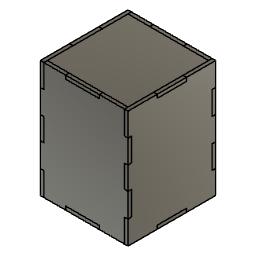
box v1 (1) (Autodesk Fusion 360 design; units mm, degrees)
Autodesk Fusion 360 part; units mm, degrees
sketch "base" plane through (0, 0, 0) normal (0, 0, 1) x (1, 0, 0)
  line L0 (37.5, 37.5) -> (-37.5, 37.5)
  line L1 (-37.5, 37.5) -> (-37.5, -37.5)
  line L2 (-37.5, -37.5) -> (37.5, -37.5)
  line L3 (37.5, -37.5) -> (37.5, 37.5)
  line L4 (37.5, 37.5) -> (-37.5, -37.5) construction
  line L5 (-37.5, 37.5) -> (37.5, -37.5) construction
  dimension "d7" = 75
  dimension "d8" = 75
  constraint horizontal L0
  constraint perpendicular L0 L1
  constraint parallel L0 L2
  constraint parallel L1 L3
  constraint coincident L4 origin
  constraint coincident L5 origin
  measures "d7" distance of L1.end L2.end
  measures "d8" distance of L0.end L1.end
extrude "Extrude1" add sketch "base" along normal blind 3 makes body 1
sketch "Sketch3" plane through (0, -37.5, 0) normal (0, -1, 0) x (1, 0, 0)
  line L0 (-37.5, 0) -> (37.5, 0)
  line L1 (37.5, 0) -> (37.5, 3)
  line L2 (37.5, 3) -> (-37.5, 3)
  line L3 (-37.5, 3) -> (-37.5, 0)
  line L4 (-37.5, 0) -> (37.5, 0)
  line L5 (37.5, 0) -> (37.5, 100)
  line L6 (37.5, 100) -> (-37.5, 100)
  line L7 (-37.5, 100) -> (-37.5, 0)
  line L8 (-15.7952, 3) -> (13, 3)
  line L9 (13, 3) -> (13, 0)
  line L10 (13, 0) -> (-15.7952, 0)
  line L11 (-15.7952, 0) -> (-15.7952, 3)
  dimension "d11" = 100
  constraint perpendicular L4 L5
  constraint parallel L4 L6
  constraint parallel L5 L7
  constraint coincident L0.end L1.start
  constraint perpendicular L1 L4
  constraint coincident L0.start L3.end
  constraint horizontal L8
  constraint vertical L9
  constraint horizontal L10
  constraint vertical L11
  constraint coincident L4 L9.end
  constraint coincident L2 L8.start
  measures "d11" distance of L0.start L6.end
extrude "Extrude3" add sketch "Sketch3" against normal blind 3 separate body contours L0 L2 L3 L4 L7 L11 | L2 L5 L6 L7 L8 | L0 L1 L2 L4 L5 L9 makes body 2
extrude "Extrude4" add 1 faces at (4.3333, -34.5, 67.6667) along direction (0, -1, 0) blind 3 from surface at -72 separate body on bodies 2 makes body 3
combine "Combine1" operation cut target body 1 tool bodies 3 2 keep tools
sketch "Sketch5" plane through (-37.5, 0, 0) normal (-1, 0, 0) x (0, -1, 0)
  line L0 (34.5, 0) -> (34.5, 3)
  line L1 (34.5, 3) -> (-34.5, 3)
  line L2 (-34.5, 3) -> (-34.5, 0)
  line L3 (-34.5, 0) -> (34.5, 0)
  line L4 (-37.5, 100) -> (-37.5, 0)
  line L5 (-37.5, 0) -> (-34.5, 0)
  line L6 (-34.5, 0) -> (-34.5, 100)
  line L7 (-34.5, 100) -> (-37.5, 100)
  line L8 (37.5, 0) -> (37.5, 100)
  line L9 (37.5, 100) -> (34.5, 100)
  line L10 (34.5, 100) -> (34.5, 0)
  line L11 (34.5, 0) -> (37.5, 0)
  line L12 (-37.5, 100) -> (37.5, 100)
  line L13 (37.5, 100) -> (37.5, 0)
  line L14 (37.5, 0) -> (-37.5, 0)
  line L15 (-37.5, 0) -> (-37.5, 100)
  line L16 (-37.5, 80) -> (-34.5, 80)
  line L17 (-34.5, 80) -> (-34.5, 60)
  line L18 (-34.5, 60) -> (-37.5, 60)
  line L19 (-37.5, 60) -> (-37.5, 80)
  line L20 (-37.5, 56.4805) -> (-37.5, 40)
  line L21 (34.5, 80) -> (37.5, 80)
  line L22 (37.5, 80) -> (37.5, 60)
  line L23 (37.5, 60) -> (34.5, 60)
  line L24 (34.5, 60) -> (34.5, 80)
  line L25 (34.5, 20) -> (37.5, 20)
  line L26 (37.5, 20) -> (37.5, 40)
  line L27 (37.5, 40) -> (34.5, 40)
  line L28 (34.5, 40) -> (34.5, 20)
  line L29 (12.5, 3) -> (-12.5, 3)
  line L30 (-12.5, 3) -> (-12.5, 0)
  line L31 (-12.5, 0) -> (12.5, 0)
  line L32 (12.5, 0) -> (12.5, 3)
  line L33 (37.5, 40.56) -> (34.5, 40.56)
  line L34 (34.5, 40.56) -> (34.5, 25)
  line L35 (34.5, 25) -> (37.5, 25)
  line L36 (37.5, 25) -> (37.5, 40.56)
  line L37 (-37.5, 39.7052) -> (-34.5, 39.7052)
  line L38 (-34.5, 39.7052) -> (-34.5, 20)
  line L39 (-34.5, 20) -> (-37.5, 20)
  line L40 (-37.5, 20) -> (-37.5, 39.7052)
  dimension "d25" = 20
  dimension "d26" = 20
  dimension "d28" = 20
  dimension "d31" = 20
  dimension "d33" = 25
  dimension "d36" = 25
  dimension "d37" = 20
  dimension "d39" = 20
  dimension "d40" = 20
  dimension "d41" = 20
  constraint horizontal L12
  constraint vertical L13
  constraint horizontal L14
  constraint vertical L15
  constraint coincident L8.start L11.end
  constraint coincident L4.start L7.end
  constraint horizontal L16
  constraint vertical L17
  constraint horizontal L18
  constraint vertical L19
  constraint coincident L6 L17.end
  constraint coincident L15 L16.start
  constraint vertical L20
  constraint coincident L4 L20.end
  constraint horizontal L21
  constraint vertical L22
  constraint horizontal L23
  constraint vertical L24
  constraint coincident L13 L22.end
  constraint coincident L10 L21.start
  constraint horizontal L25
  constraint vertical L26
  constraint horizontal L27
  constraint vertical L28
  constraint coincident L8 L26.end
  constraint coincident L10 L25.start
  constraint horizontal L29
  constraint vertical L30
  constraint horizontal L31
  constraint vertical L32
  constraint coincident L14 L30.end
  constraint coincident L1 L29.start
  constraint horizontal L33
  constraint vertical L34
  constraint horizontal L35
  constraint vertical L36
  constraint coincident L10 L34.end
  constraint coincident L13 L33.start
  constraint horizontal L37
  constraint vertical L38
  constraint horizontal L39
  constraint vertical L40
  constraint coincident L6 L38.end
  constraint coincident L20 L37.start
  measures "d25" distance of L8.end L21.end
  measures "d26" distance of L21.start L23.end
  measures "d28" distance of L4.start L16.start
  measures "d31" distance of L16.start L18.end
  measures "d33" distance of L8.start L31.end
  measures "d36" distance of L29.start L29.end
  measures "d37" distance of L22.end L26.end
  measures "d39" distance of L18.end L20.end
  measures "d40" distance of L20.end L39.end
  measures "d41" distance of L25.end L26.end
extrude "Extrude5" add sketch "Sketch5" against normal blind 3 separate body contours L0 L1 L3 L10 L14 L32 | L0 L8 L10 L11 L13 L14 L25 | L1 L6 L10 L12 L17 L24 L28 L29 L34 L38 | L1 L2 L3 L6 L14 L30 | L2 L4 L5 L6 L14 L15 L39 | L8 L10 L13 L23 L33 | L4 L6 L15 L18 L20 L37 | L8 L9 L10 L12 L13 L21 | L4 L6 L7 L12 L15 L16 makes body 4
extrude "Extrude6" add 1 faces at (-34.5, -4.1667, 27.5684) along direction (-1, 0, 0) blind 3 from surface at -72 separate body on bodies 4 makes body 5
combine "Combine2" operation cut target body 2 tool bodies 5 4 keep tools
sketch "Sketch7" plane through (0, 37.5, 0) normal (0, 1, 0) x (-1, 0, 0)
  line L0 (-13, 3) -> (15.7952, 3)
  line L1 (15.7952, 3) -> (15.7952, 0)
  line L2 (15.7952, 0) -> (37.5, 0)
  line L3 (37.5, 0) -> (37.5, 100)
  line L4 (37.5, 100) -> (-37.5, 100)
  line L5 (-37.5, 100) -> (-37.5, 0)
  line L6 (-37.5, 0) -> (-13, 0)
  line L7 (-13, 0) -> (-13, 3)
combine "Combine3" operation cut target body 3 tool bodies 5 4 keep tools
sketch "Sketch8" plane through (0, -37.5, 0) normal (0, -1, 0) x (1, 0, 0)
  line L0 (-34.5, 20) -> (-34.5, 0)
  line L1 (-34.5, 0) -> (-15.7952, 0)
  line L2 (-15.7952, 0) -> (-15.7952, 3)
  line L3 (-15.7952, 3) -> (13, 3)
  line L4 (13, 3) -> (13, 0)
  line L5 (13, 0) -> (34.5, 0)
  line L6 (34.5, 0) -> (34.5, 20)
  line L7 (34.5, 20) -> (37.5, 20)
  line L8 (37.5, 20) -> (37.5, 40.56)
  line L9 (37.5, 40.56) -> (34.5, 40.56)
  line L10 (34.5, 40.56) -> (34.5, 60)
  line L11 (34.5, 60) -> (37.5, 60)
  line L12 (37.5, 60) -> (37.5, 80)
  line L13 (37.5, 80) -> (34.5, 80)
  line L14 (34.5, 80) -> (34.5, 100)
  line L15 (34.5, 100) -> (-34.5, 100)
  line L16 (-34.5, 100) -> (-34.5, 80)
  line L17 (-34.5, 80) -> (-37.5, 80)
  line L18 (-37.5, 80) -> (-37.5, 60)
  line L19 (-37.5, 60) -> (-34.5, 60)
  line L20 (-34.5, 60) -> (-34.5, 40.56)
  line L21 (-34.5, 40.56) -> (-37.5, 40.56)
  line L22 (-37.5, 40.56) -> (-37.5, 20)
  line L23 (-37.5, 20) -> (-34.5, 20)
sketch "Sketch9" plane through (0, -37.5, 50) normal (0, -1, 0) x (1, 0, 0)
combine "Combine4" operation cut target body 1 tool bodies 4 5 keep tools
extrude "Extrude7" add 1 faces at (-11.5, 4.1667, 3) along direction (0, 0, -1) blind 3 from surface at -97 separate body on bodies 1 makes body 6
sketch "right-dxf" plane through (37.5, 0, 0) normal (1, 0, 0) x (0, 1, 0)
  line L0 (34.5, 20) -> (34.5, 39.7052)
  line L1 (34.5, 39.7052) -> (37.5, 39.7052)
  line L2 (37.5, 39.7052) -> (37.5, 60)
  line L3 (37.5, 60) -> (34.5, 60)
  line L4 (34.5, 60) -> (34.5, 80)
  line L5 (34.5, 80) -> (37.5, 80)
  line L6 (37.5, 80) -> (37.5, 100)
  line L7 (37.5, 100) -> (-37.5, 100)
  line L8 (-37.5, 100) -> (-37.5, 80)
  line L9 (-37.5, 80) -> (-34.5, 80)
  line L10 (-34.5, 80) -> (-34.5, 60)
  line L11 (-34.5, 60) -> (-37.5, 60)
  line L12 (-37.5, 60) -> (-37.5, 40.56)
  line L13 (-37.5, 40.56) -> (-34.5, 40.56)
  line L14 (-34.5, 40.56) -> (-34.5, 20)
  line L15 (-34.5, 20) -> (-37.5, 20)
  line L16 (-37.5, 20) -> (-37.5, 0)
  line L17 (-37.5, 0) -> (-12.5, 0)
  line L18 (-12.5, 0) -> (-12.5, 3)
  line L19 (-12.5, 3) -> (12.5, 3)
  line L20 (12.5, 3) -> (12.5, 0)
  line L21 (12.5, 0) -> (37.5, 0)
  line L22 (37.5, 0) -> (37.5, 20)
  line L23 (37.5, 20) -> (34.5, 20)
sketch "base-dxf" plane through (0, 0, 3) normal (0, 0, 1) x (-1, 0, 0)
  line L0 (-34.5, 34.5) -> (-34.5, 12.5)
  line L1 (-34.5, 12.5) -> (-37.5, 12.5)
  line L2 (-37.5, 12.5) -> (-37.5, -12.5)
  line L3 (-37.5, -12.5) -> (-34.5, -12.5)
  line L4 (-34.5, -12.5) -> (-34.5, -34.5)
  line L5 (-34.5, -34.5) -> (-13, -34.5)
  line L6 (-13, -34.5) -> (-13, -37.5)
  line L7 (-13, -37.5) -> (15.7952, -37.5)
  line L8 (15.7952, -37.5) -> (15.7952, -34.5)
  line L9 (15.7952, -34.5) -> (34.5, -34.5)
  line L10 (34.5, -34.5) -> (34.5, -12.5)
  line L11 (34.5, -12.5) -> (37.5, -12.5)
  line L12 (37.5, -12.5) -> (37.5, 12.5)
  line L13 (37.5, 12.5) -> (34.5, 12.5)
  line L14 (34.5, 12.5) -> (34.5, 34.5)
  line L15 (34.5, 34.5) -> (15.7952, 34.5)
  line L16 (15.7952, 34.5) -> (15.7952, 37.5)
  line L17 (15.7952, 37.5) -> (-13, 37.5)
  line L18 (-13, 37.5) -> (-13, 34.5)
  line L19 (-13, 34.5) -> (-34.5, 34.5)
sketch "back-dxf" plane through (0, 34.5, 0) normal (0, -1, 0) x (1, 0, 0)
  line L0 (-34.5, 20) -> (-34.5, 0)
  line L1 (-34.5, 0) -> (-15.7952, 0)
  line L2 (-15.7952, 0) -> (-15.7952, 3)
  line L3 (-15.7952, 3) -> (13, 3)
  line L4 (13, 3) -> (13, 0)
  line L5 (13, 0) -> (34.5, 0)
  line L6 (34.5, 0) -> (34.5, 20)
  line L7 (34.5, 20) -> (37.5, 20)
  line L8 (37.5, 20) -> (37.5, 39.7052)
  line L9 (37.5, 39.7052) -> (34.5, 39.7052)
  line L10 (34.5, 39.7052) -> (34.5, 60)
  line L11 (34.5, 60) -> (37.5, 60)
  line L12 (37.5, 60) -> (37.5, 80)
  line L13 (37.5, 80) -> (34.5, 80)
  line L14 (34.5, 80) -> (34.5, 100)
  line L15 (34.5, 100) -> (-34.5, 100)
  line L16 (-34.5, 100) -> (-34.5, 80)
  line L17 (-34.5, 80) -> (-37.5, 80)
  line L18 (-37.5, 80) -> (-37.5, 60)
  line L19 (-37.5, 60) -> (-34.5, 60)
  line L20 (-34.5, 60) -> (-34.5, 39.7052)
  line L21 (-34.5, 39.7052) -> (-37.5, 39.7052)
  line L22 (-37.5, 39.7052) -> (-37.5, 20)
  line L23 (-37.5, 20) -> (-34.5, 20)
equation "length = 75 mm" comment "box length"
equation "width = 75 mm" comment "box width"
equation "height = 100 mm" comment "box height"
equation "hole = 60 mm" comment "opening"
equation "t = 3 mm" comment "plywood thickness"
equation "d7 = length"
equation "d8 = width"
equation "d9 = t"
equation "d11 = height"
equation "slotL = length / 3" comment "size of slot @length"
equation "slotW = width / 3" comment "size of slot @width"
equation "d18 = -t"
equation "slotH = height / 5" comment "size of slot @height"
equation "d22 = -t"
equation "d25 = slotH"
equation "d26 = d25"
equation "d27 = d26"
equation "d28 = slotH"
equation "d31 = d28"
equation "d33 = slotW"
equation "d36 = slotW"
equation "d37 = d26"
equation "d39 = d28"
equation "d40 = d28"
equation "d41 = d25"
equation "d42 = -t"
equation "d45 = -t"
equation "d48 = -t"
named bodies: "base", "front", "back"
